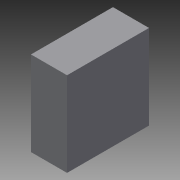
# Autodesk Inventor part: solenoid_dvr
Saved by Autodesk Inventor 2015 (Build 190159000, 159)
## iProperties
Created: 2015-10-09
Part Number: solenoid_dvr
Material: Generic
Description: insert part description/title
Document SubType Name: Modeling
Designer: c3132704
Density: 1 g/cm^3
Appearance: Default
Author: c3132704
Part Category: insert part category here and press enter to fill value
Autodesk Inventor part; units mm, degrees
ref_plane "YZ Plane" through (0, 0, 0) normal (1, 0, 0) x (0, 1, 0)
ref_plane "XZ Plane" through (0, 0, 0) normal (0, 1, 0) x (-1, 0, 0)
ref_plane "XY Plane" through (0, 0, 0) normal (0, 0, 1) x (1, 0, 0)
sketch "Sketch1" plane through (0, 0, 0) normal (1, 0, 0) x (0, 1, 0)
  line L0 (32.6696, 26.5124) -> (-46.8304, 26.5124)
  line L1 (-46.8304, 26.5124) -> (-46.8304, -55.4876)
  line L2 (-46.8304, -55.4876) -> (32.6696, -55.4876)
  line L3 (32.6696, -55.4876) -> (32.6696, 26.5124)
  point P0 (0, 0)
  dimension "d0" = 82
  dimension "d1" = 79.5
  constraints: 8 end point, 2 parallel, 1 horizontal, 1 perpendicular
  measures "d0" distance of L2.end L0.start
  measures "d1" distance of L0.start L0.end
extrude "Extrusion1" add sketch "Sketch1" along normal blind 35
body "Solid1"
